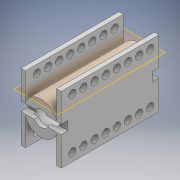
# Autodesk Inventor part: slider-magnet-carrier
Saved by Autodesk Inventor 2018 (Build 220112000, 112)
## iProperties
Created: 2025-08-23
Part Number: slider-magnet-carrier
Material: Generic
Document SubType Name: Modeling
Designer: neo
Density: 1 g/cm^3
Appearance: Default
Author: neo
Autodesk Inventor part; units mm, degrees
ref_plane "YZ Plane" through (0, 0, 0) normal (1, 0, 0) x (0, 1, 0)
ref_plane "XZ Plane" through (0, 0, 0) normal (0, 1, 0) x (-1, 0, 0)
ref_plane "XY Plane" through (0, 0, 0) normal (0, 0, 1) x (1, 0, 0)
sketch "Sketch1" plane through (0, 0, 0) normal (0, 1, 0) x (-1, 0, 0)
  line L0 (13.1536, 14.8262) -> (11.1536, 14.8262)
  line L1 (11.1536, 14.8262) -> (11.1536, -15.1738)
  line L2 (11.1536, -15.1738) -> (13.1536, -15.1738)
  line L3 (13.1536, -15.1738) -> (13.1536, 14.8262)
  line L4 (-2.8464, 14.8262) -> (-4.8464, 14.8262)
  line L5 (-4.8464, 14.8262) -> (-4.8464, -15.1738)
  line L6 (-4.8464, -15.1738) -> (-2.8464, -15.1738)
  line L7 (-2.8464, -15.1738) -> (-2.8464, 14.8262)
  line L8 (11.4509, -0.1738) -> (-13.3196, -0.1738)
  line L9 (4.1536, 20.4248) -> (4.1536, -20.4682)
  circle A0 centre (4.1536, -0.1738) radius 5.5
  circle A1 centre (4.1536, -0.1738) radius 7.5
  point P0 (0, 0)
  dimension "d2" = 14
  dimension "d3" = 2
  dimension "d4" = 2
  dimension "d5" = 11
  dimension "d6" = 15
  constraints: 20 end point, 4 parallel, 3 horizontal, 2 centre point, 2 coincident, 2 perpendicular, 2 point on line, 1 collinear, 1 vertical, 4 other
  measures "d2" distance between parallel lines of L7 L1
  measures "d3" distance between parallel lines of L1 L3
  measures "d4" radial gap between concentric circles of A0 A1
  measures "d5" diameter of A0
  measures "d6" distance from line of A1.centre L0
extrude "Extrusion1" add sketch "Sketch1" along normal blind 44 contours L3 L2 L1 A1 L0 | A1 L1 | L1 L8 A0 L9 A1 | L1 A1 L9 A0 L8 | L9 A0 L8 L7 A1 | A1 L8 L5 L4 L7 | L7 L8 A1 | A1 L7 L8 A0 L9 | L7 A1 L8 | A1 L7 L6 L5 L8
sketch "Sketch2" plane through (4.8464, 0, 14.8262) normal (1, 0, 0) x (0, 0, -1)
  line L0 (14.8262, 0) -> (14.8262, 49.2692)
  line L1 (3.5, 48.2793) -> (3.5, -5.9843)
  circle A0 centre (3.5, 40) radius 1.65
  line L2 (0, 0) -> (0, 44) projected
  line L3 (0, 44) -> (30, 44) projected
  circle A1 centre (3.5, 35) radius 1.65
  circle A2 centre (3.5, 30) radius 1.65
  circle A3 centre (3.5, 25) radius 1.65
  circle A4 centre (3.5, 20) radius 1.65
  circle A5 centre (3.5, 15) radius 1.65
  circle A6 centre (3.5, 10) radius 1.65
  circle A7 centre (3.5, 5) radius 1.65
  circle A8 centre (26.1523, 40) radius 1.65
  line L4 (29.6523, 0) -> (29.6523, 44)
  circle A9 centre (26.1523, 35) radius 1.65
  circle A10 centre (26.1523, 30) radius 1.65
  circle A11 centre (26.1523, 25) radius 1.65
  circle A12 centre (26.1523, 20) radius 1.65
  circle A13 centre (26.1523, 15) radius 1.65
  circle A14 centre (26.1523, 10) radius 1.65
  circle A15 centre (26.1523, 5) radius 1.65
  circle A16 centre (3.5, 0) radius 1.65
  circle A17 centre (26.1523, 0) radius 1.65
  point P0 (26.1523, 48.2793)
  dimension "d9" = 3.5
  dimension "d10" = 3.3
  dimension "d11" = 4
  dimension "d14" = 5
  dimension "d26" = 5
  constraints: 18 centre point, 12 symmetric about line, 6 end point, 4 vertical, 1 point on line, 25 other
  measures "d9" distance between parallel lines of L2 L1
  measures "d10" diameter of A0
  measures "d11" distance from line of L3 A0.centre
  measures "d14" distance of A0.centre A1.centre
  measures "d26" distance of A7.centre A16.centre
extrude "Extrusion2" cut sketch "Sketch2" against normal through all contours A0 L1 | A7 L1 | L1 A7 | A6 L1 | L1 A6 | A5 L1 | L1 A5 | A4 L1 | L1 A4 | A3 L1 | L1 A3 | A2 L1 | L1 A2 | A1 L1 | L1 A1 | L1 A0 | A8 | A9 | A10 | A11 | A12 | A13 | A14 | A15
sketch "Sketch3" plane through (0, 0, 0) normal (0, -1, 0) x (1, 0, 0)
  circle A0 centre (-4.1536, -0.1738) radius 5.5 projected
  circle A1 centre (-4.1536, -0.1738) radius 3.5
  point P0 (0, 0)
  dimension "d21" = 2
  constraints: 1 centre point, 1 coincident
  measures "d21" radial gap between concentric circles of A1 A0
extrude "Extrusion3" add sketch "Sketch3" against normal blind 1.8
sketch "Sketch4" plane through (4.8464, 0, 14.8262) normal (1, 0, 0) x (0, 0, -1)
  line L0 (14.8262, 0) -> (14.8262, 46.2334)
  line L1 (0, 0) -> (12.3074, 0) projected
  line L2 (12.8262, 0) -> (16.8262, 0)
  line L3 (16.8262, 0) -> (16.8262, 3)
  line L4 (16.8262, 3) -> (12.8262, 3)
  line L5 (12.8262, 3) -> (12.8262, 0)
  line L6 (12.8262, 41) -> (16.8262, 41)
  line L7 (16.8262, 41) -> (16.8262, 44)
  line L8 (16.8262, 44) -> (12.8262, 44)
  line L9 (12.8262, 44) -> (12.8262, 41)
  dimension "d32" = 4
  dimension "d33" = 3
  dimension "d34" = 4
  dimension "d35" = 3
  constraints: 18 end point, 4 parallel, 2 horizontal, 2 perpendicular, 1 point on line, 1 vertical, 2 other
  measures "d32" distance between parallel lines of L3 L5
  measures "d33" distance of L4.end L2.start
  measures "d34" distance of L7.end L8.end
  measures "d35" distance of L8.end L6.start
extrude "Extrusion4" cut sketch "Sketch4" against normal through all
ref_plane "Work Plane1" through (-4.1536, 0, 7.3262) normal (0, 0, 1) x (1, 0, 0)
body "Solid1"
